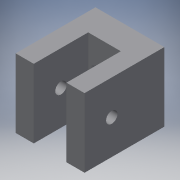
# Autodesk Inventor part: YPulleySupportHolder
Saved by Autodesk Inventor 2019 (Build 230136000, 136)
## iProperties
Created: 2019-08-19
Part Number: YPulleySupportHolder
Material: Generic
Document SubType Name: Modeling
Designer: Bruno
Density: 1 g/cm^3
Appearance: Default
Author: Bruno
Autodesk Inventor part; units mm, degrees
ref_plane "YZ Plane" through (0, 0, 0) normal (1, 0, 0) x (0, 1, 0)
ref_plane "XZ Plane" through (0, 0, 0) normal (0, 1, 0) x (-1, 0, 0)
ref_plane "XY Plane" through (0, 0, 0) normal (0, 0, 1) x (1, 0, 0)
sketch "Sketch1" plane through (0, 0, 0) normal (0, 0, 1) x (1, 0, 0)
  line L0 (-13.1198, 5.618) -> (5.8802, 5.618)
  line L1 (5.8802, 5.618) -> (5.8802, -13.382)
  line L2 (5.8802, -13.382) -> (-13.1198, -13.382)
  line L3 (-13.1198, -13.382) -> (-13.1198, 5.618)
  point P0 (0, 0)
  dimension "d0" = 19
  dimension "d1" = 19
  constraints: 8 end point, 2 parallel, 1 horizontal, 1 perpendicular
  measures "d0" distance of L0.end L1.end
  measures "d1" distance of L0.start L0.end
extrude "Extrusion1" add sketch "Sketch1" along normal blind 7
sketch "Sketch2" plane through (0, 0, 7) normal (0, 0, 1) x (1, 0, 0)
  line L0 (5.8802, 5.618) -> (-13.1198, 5.618) projected
  line L1 (-13.1198, 5.618) -> (-13.1198, -13.382) projected
  line L2 (-13.1198, -13.382) -> (5.8802, -13.382) projected
  line L3 (5.8802, -13.382) -> (5.8802, 5.618) projected
  line L4 (-13.1198, -13.382) -> (5.8802, -13.382) projected
  line L5 (-8.1198, -13.382) -> (-8.1198, 5.618)
  line L6 (5.8802, 5.618) -> (-13.1198, 5.618) projected
  line L7 (0.8802, -13.382) -> (0.8802, 5.618)
  line L8 (-13.1198, 3.1934) -> (-8.1198, 3.1934) construction
  line L9 (-8.1198, 3.1934) -> (0.8802, 3.1934) construction
  line L10 (0.8802, 3.1934) -> (5.8802, 3.1934) construction
  point P0 (0, 0)
  dimension "d4" = 9
  constraints: 10 end point, 10 point on line, 2 perpendicular, 1 collinear, 1 parallel
  measures "d4" distance of L8.end L9.end
extrude "Extrusion2" add sketch "Sketch2" along normal blind 15 contours L3 L2 L7 L0 | L5 L2 L1 L0
sketch "Sketch3" plane through (0, 0, 0) normal (0, 0, -1) x (-1, 0, 0)
  circle A0 centre (3.6198, -3.882) radius 2.125
  line L0 (13.1198, 5.618) -> (-5.8802, 5.618) projected
  line L1 (13.1198, -13.382) -> (8.1198, -13.382) projected
  line L2 (-5.8802, 5.618) -> (13.1198, -13.382) construction
  line L3 (13.1198, 5.618) -> (-5.8802, -13.382) construction
  point P0 (0, 0)
  dimension "d7" = 4.25
  constraints: 4 end point, 2 coincident, 1 centre point, 1 midpoint
  measures "d7" diameter of A0
extrude "Extrusion3" cut sketch "Sketch3" against normal up to next
sketch "Sketch4" plane through (5.8802, -13.382, 0) normal (1, 0, 0) x (0, 0, -1)
  circle A0 centre (-14.5, 9.5) radius 1.575
  line L0 (-7, 0) -> (-7, 19) projected
  line L1 (-7, 0) -> (-22, 0) projected
  line L2 (-22, 0) -> (-7, 19) construction
  line L3 (-22, 0) -> (-22, 19) projected
  line L4 (-7, 0) -> (-22, 19) construction
  point P0 (0, 13.382)
  dimension "d10" = 3.15
  constraints: 4 end point, 1 centre point, 1 coincident, 1 midpoint
  measures "d10" diameter of A0
extrude "Extrusion4" cut sketch "Sketch4" against normal through all
sketch "Sketch5" plane through (0, 0, 7) normal (0, 0, 1) x (1, 0, 0)
  line L0 (-3.6198, 0.243) -> (-0.0475, -1.8195)
  line L1 (-0.0475, -1.8195) -> (-0.0475, -5.9445)
  line L2 (-0.0475, -5.9445) -> (-3.6198, -8.007)
  line L3 (-3.6198, -8.007) -> (-7.1922, -5.9445)
  line L4 (-7.1922, -5.9445) -> (-7.1922, -1.8195)
  line L5 (-7.1922, -1.8195) -> (-3.6198, 0.243)
  circle A0 centre (-3.6198, -3.882) radius 2.125 projected
  point P0 (0, 0)
  dimension "d13" = 8.25
  constraints: 12 end point, 1 coincident, 1 vertical, 13 other
  measures "d13" distance of L2.end L0.start
extrude "Extrusion5" cut sketch "Sketch5" against normal blind 3.2
body "Solid1"
